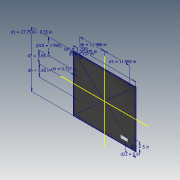
# Autodesk Inventor part: FLUGGER LOWER BACK COVER
Saved by Autodesk Inventor 2020.3 (Build 243373000, 373)
## iProperties
RuleStatus: InUse
AfterDocSave0: file://Part Number Cleaner
Created: 2020-01-03
Material: ALUMINUM, 6061-T651
Vendor: HHMI: JRC - ID&F
Document SubType Name: Modeling
Designer: arnoldj
Density: 2.7 g/cm^3
Appearance: Anodized - Light Gray
DESIGN DEPARTMENT: HHMI: JRC - ID&F
ALTERED ITEM PART NUMBER: N/A
ALTERED ITEM VENDOR: N/A
ALTERED ITEM DESCRIPTION: N/A
Author: arnoldj
Revision Number: 0
Autodesk Inventor part; units mm, degrees
ref_plane "YZ Plane" through (0, 0, 0) normal (1, 0, 0) x (0, 1, 0)
ref_plane "XZ Plane" through (0, 0, 0) normal (0, 1, 0) x (-1, 0, 0)
ref_plane "XY Plane" through (0, 0, 0) normal (0, 0, 1) x (1, 0, 0)
sketch "Sketch1" plane through (0, 0, 0) normal (0, 0, 1) x (1, 0, 0)
  line L0 (0, 483.616) -> (0, -483.616) projected
  line L1 (-541.8455, 0) -> (541.8455, 0) projected
  line L2 (387.0325, -345.44) -> (-387.0325, -345.44)
  line L3 (-387.0325, -345.44) -> (-387.0325, 345.44)
  line L4 (-387.0325, 345.44) -> (387.0325, 345.44)
  line L5 (387.0325, 345.44) -> (387.0325, -345.44)
  line L6 (387.0325, -345.44) -> (-387.0325, 345.44) construction
  line L7 (-387.0325, -345.44) -> (387.0325, 345.44) construction
  line L8 (368.3127, -326.7202) -> (-368.3127, -326.7202) construction
  line L9 (-368.3127, -326.7202) -> (-368.3127, 326.7202) construction
  line L10 (-368.3127, 326.7202) -> (368.3127, 326.7202) construction
  line L11 (368.3127, 326.7202) -> (368.3127, -326.7202) construction
  line L12 (368.3127, -326.7202) -> (-368.3127, 326.7202) construction
  line L13 (-368.3127, -326.7202) -> (368.3127, 326.7202) construction
  point P0 (0, 0)
  point P1 (-304.4952, 326.7202)
  point P2 (0, 326.7202)
  point P3 (304.4952, 326.7202)
  point P4 (-304.4952, -326.7202)
  point P5 (0, -326.7202)
  point P6 (-368.3127, 143.51)
  point P7 (-368.3127, -143.51)
  point P8 (368.3127, 143.51)
  point P9 (260.0325, -326.7202)
  point P10 (368.3127, -218.44)
  dimension "d0" = 774.065
  dimension "d1" = 690.88
  dimension "d3" = 18.7198
  dimension "d4" = 18.7198
  dimension "d5" = 304.4952
  dimension "d6" = 304.4952
  dimension "d7" = 143.51
  dimension "d8" = 143.51
  dimension "d9" = 82.5373
  dimension "d10" = 201.93
  dimension "d22" = 127
  dimension "d23" = 127
  constraints: 24 end point, 8 point on line, 6 midpoint, 4 parallel, 2 horizontal, 2 perpendicular, 1 horizontal alignment, 1 vertical alignment
  measures "d0" distance of L3.end L4.end
  measures "d1" distance of L2.end L3.end
  measures "d3" distance between parallel lines of L10 L4
  measures "d4" distance between parallel lines of L9 L3
  measures "d5" distance from line of L0 point (304.495, 326.72)
  measures "d6" distance from line of L0 point (-304.495, 326.72)
  measures "d7" distance from line of L1 point (-368.313, 143.51)
  measures "d8" distance from line of point (-368.313, -143.51) L1
  measures "d9" distance from line of point (-304.495, 326.72) L3
  measures "d10" distance from line of point (-368.313, 143.51) L4
  measures "d22" distance from line of point (368.313, -218.44) L2
  measures "d23" distance from line of point (260.033, -326.72) L5
extrude "Extrusion1" add sketch "Sketch1" against normal blind 3.175
hole "Hole1" at (-304.4952, -326.7202, 0) at (0, -326.7202, 0) at (-368.3127, 143.51, 0) at (-368.3127, -143.51, 0) at (368.3127, 143.51, 0) at (368.3127, -218.44, 0) at (260.0325, -326.7202, 0) direction (0, 0, -1) diameter 7.9375 end through all
fillet "Fillet1" radius 6.35 4 edges at (387.0325, 345.44, -1.5875) (387.0325, -345.44, -1.5875) (-387.0325, -345.44, -1.5875) (-387.0325, 345.44, -1.5875)
sketch "Sketch2" plane through (0, 0, 0) normal (0, 0, 1) x (1, 0, 0)
  line L0 (380.6825, -345.44) -> (-380.6825, -345.44) projected
  line L1 (387.0325, 345.44) -> (387.0325, -345.44) projected
  line L2 (387.0325, -345.44) -> (310.8325, -345.44)
  line L3 (387.0325, -269.24) -> (387.0325, -345.44)
  line L4 (380.6825, -345.44) -> (-380.6825, -345.44) projected
  line L5 (192.3288, -345.44) -> (192.3288, -256.54)
  line L6 (192.3288, -256.54) -> (287.5788, -256.54)
  line L7 (287.5788, -256.54) -> (287.5788, -345.44)
  line L8 (192.3288, -256.54) -> (287.5788, -345.44) construction
  line L9 (192.3288, -345.44) -> (287.5788, -256.54) construction
  line L10 (0, 483.616) -> (0, -483.616) construction
  line L11 (-541.8455, 0) -> (541.8455, 0) construction
  line L12 (192.3288, -297.815) -> (287.5788, -297.815)
  point P0 (0, 0)
  point P1 (239.9538, -300.99)
  point P2 (192.3288, -345.44)
  dimension "d28" = 239.9538
  dimension "d29" = 95.25
  dimension "d30" = 88.9
  dimension "d31" = 47.625
  constraints: 16 end point, 4 perpendicular, 4 point on line, 1 horizontal, 1 midpoint
  measures "d28" distance from line of point (239.954, -300.99) L10
  measures "d29" distance of L5.end L6.end
  measures "d30" distance of L5.start L5.end
  measures "d31" distance between parallel lines of L12 L0
extrude "Extrusion2" cut sketch "Sketch2" against normal through all contours L12 L5 L6 L7
fillet "Fillet3" radius 6.35 4 edges at (192.3288, -256.54, -1.5875) (287.5788, -256.54, -1.5875) (287.5788, -297.815, -1.5875) (192.3288, -297.815, -1.5875)
hole "Hole2" at (-304.4952, 326.7202, 0) at (0, 326.7202, 0) at (304.4952, 326.7202, 0) direction (0, 0, -1) diameter 3.2512 end through all
body "Solid1"
